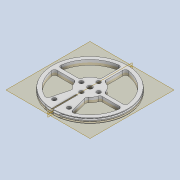
# Autodesk Inventor part: driver_wheel_1
Saved by Autodesk Inventor 2020 (Build 240168000, 168)
## iProperties
Created: 2021-08-04
Part Number: driver_wheel_1
Material: Generic
Document SubType Name: Modeling
Designer: Shuang Peng
Density: 1 g/cm^3
Appearance: Default
Author: Shuang Peng
Autodesk Inventor part; units mm, degrees
ref_plane "YZ Plane" through (0, 0, 0) normal (1, 0, 0) x (0, 1, 0)
ref_plane "XZ Plane" through (0, 0, 0) normal (0, 1, 0) x (-1, 0, 0)
ref_plane "XY Plane" through (0, 0, 0) normal (0, 0, 1) x (1, 0, 0)
sketch "Sketch1" plane through (0, 0, 0) normal (0, 1, 0) x (-1, 0, 0)
  circle A0 centre (0, 0) radius 30
  dimension "d0" = 60
  constraints: 1 centre point, 1 coincident
  measures "d0" diameter of A0
extrude "Extrusion1" add sketch "Sketch1" along normal blind 2
sketch "Sketch2" plane through (0, 0, 0) normal (1, 0, 0) x (0, 1, 0)
  line L0 (0, 30) -> (2, 30) projected
  line L1 (2, -30) -> (2, 30) projected
  line L2 (2, 30) -> (2, 31)
  line L3 (2, 31) -> (1, 30)
  line L4 (0, -30) -> (0, 30) projected
  line L5 (0, 30) -> (0, 31)
  line L6 (0, 31) -> (1, 30)
  line L7 (0, 0) -> (2, 0)
  dimension "d3" = 1
  dimension "d4" = 1
  constraints: 10 end point, 2 midpoint, 2 vertical
  measures "d3" distance of L0.end L2.end
  measures "d4" distance of L0.start L5.end
revolve "Revolution1" add sketch "Sketch2" angle 360 about axis through (0, 0, 0) along (0, 1, 0) contours L5 L6 L0 | L3 L2 L0
sketch "Sketch3" plane through (0, 2, 0) normal (0, 1, 0) x (1, 0, 0)
  circle A0 centre (0, 0) radius 1.5
  dimension "d6" = 3
  constraints: 1 centre point, 1 coincident
  measures "d6" diameter of A0
extrude "Extrusion2" cut sketch "Sketch3" against normal blind 2
sketch "Sketch4" plane through (0, 2, 0) normal (0, 1, 0) x (1, 0, 0)
  circle A0 centre (0, 0) radius 1.5 projected
  circle A1 centre (0, 0) radius 31 projected
  circle A2 centre (0, 0) radius 1.5 projected
  line L0 (0, 0) -> (0, -31)
  circle A3 centre (0, 0) radius 31 projected
  line L1 (0, -51) -> (0, -11) construction
  line L2 (0.5, -51) -> (0.5, -11)
  line L3 (-0.5, -11) -> (-0.5, -51)
  arc A4 (-0.5, -51) -> (0.5, -51) centre (0, -51) ccw
  arc A5 (0.5, -11) -> (-0.5, -11) centre (0, -11) ccw
  point P0 (-0.5, -30.996)
  point P1 (0.5, -30.996)
  dimension "d9" = 20
  dimension "d10" = 1
  constraints: 10 end point, 4 point on circle, 4 tangent, 2 centre point, 1 midpoint, 1 parallel, 1 point on line, 1 vertical, 1 vertical alignment, 1 other
  measures "d9" distance of L0.end L1.end
  measures "d10" diameter of A5
extrude "Extrusion3" cut sketch "Sketch4" against normal blind 2 contours L3 A5 L0 A1 | A1 L0 A5 L2
ref_plane "Work Plane1" through (0, 2, 30.996) normal (1, 0, 0) x (0, 0, -1)
sketch "Sketch5" plane through (-0.5, 2, 30.996) normal (1, 0, 0) x (0, 0, -1)
  line L0 (0, -2) -> (1.0001, -1) projected
  line L1 (19.996, -2) -> (0, -2) projected
  line L2 (19.996, 0) -> (19.996, -2) projected
  line L3 (0, 0) -> (19.996, 0) projected
  line L4 (1.0001, -1) -> (0, 0) projected
  line L5 (60.996, -1) -> (1.0001, -1) projected
  line L6 (1.0001, -1) -> (2.0001, -1)
  line L7 (0, 0) -> (19.996, 0) projected
  line L8 (2.0001, -1) -> (0, 0)
  line L9 (19.996, -2) -> (0, -2) projected
  line L10 (2.0001, -1) -> (0, -2)
  point P0 (30.996, -2)
  dimension "d13" = 1
  constraints: 6 end point, 1 parallel
  measures "d13" distance of L0.end L6.end
extrude "Extrusion4" cut sketch "Sketch5" against normal blind 12 contours L0 L5 L10 | L4 L8 L5
mirror "Mirror1" about plane through (0, 2, 30.996) normal (1, 0, 0) of "Extrusion4"
sketch "Sketch6" plane through (0, 2, 0) normal (0, 1, 0) x (1, 0, 0)
  line L0 (0.5, -11) -> (0.5, -30.996) projected
  arc A0 (0.5, -30.996) -> (-0.5, -30.996) centre (0, 0) ccw projected
  line L1 (-0.5, -30.996) -> (-0.5, -11) projected
  arc A1 (0.5, -11) -> (-0.5, -11) centre (0, -11) ccw projected
  circle A2 centre (0, 0) radius 1.5 projected
  line L2 (0, 0) -> (-6, 0)
  line L3 (-6, 0) -> (-6, -23)
  circle A3 centre (-6, -23) radius 1.6
  dimension "d16" = 6
  dimension "d17" = 23
  dimension "d18" = 3.2
  constraints: 4 end point, 1 centre point, 1 coincident, 1 horizontal, 1 perpendicular
  measures "d16" distance of L2.start L2.end
  measures "d17" distance of L2.end L3.end
  measures "d18" diameter of A3
extrude "Extrusion5" cut sketch "Sketch6" against normal blind 12 contours A3
mirror "Mirror2" about plane through (0, 2, 30.996) normal (1, 0, 0) of "Extrusion5"
ref_plane "Work Plane2" through (0, 2, 0) normal (0, 1, 0) x (1, 0, 0)
mirror "Mirror3" about plane through (0, 2, 0) normal (0, 1, 0) of "Extrusion1", "Revolution1", "Extrusion2", "Extrusion3", "Extrusion4", "Mirror1", "Extrusion5", "Mirror2"
chamfer "Chamfer1" distance 0.5 angle 45 3 edges at (0, 2, -31) (0, 4, -31) (0, 0, -31)
sketch "Sketch7" plane through (0, 4, 0) normal (0, 1, 0) x (1, 0, 0)
  line L0 (0, 0) -> (-7, 0)
  circle A0 centre (-7, 0) radius 1.6
  circle A1 centre (0, -7) radius 1.6
  circle A2 centre (7, 0) radius 1.6
  circle A3 centre (0, 7) radius 1.6
  dimension "d25" = 7
  dimension "d26" = 3.2
  dimension "d29" = 360
  constraints: 4 centre point, 2 end point, 1 coincident, 1 horizontal, 9 other
  measures "d25" distance of L0.start L0.end
  measures "d26" diameter of A0
extrude "Extrusion6" cut sketch "Sketch7" against normal blind 12
sketch "Sketch8" plane through (0, 4, 0) normal (0, 1, 0) x (1, 0, 0)
  circle A0 centre (7, 0) radius 1.6 projected
  circle A1 centre (0, 7) radius 1.6 projected
  circle A2 centre (0, -7) radius 1.6 projected
  circle A3 centre (-7, 0) radius 1.6 projected
  arc A4 (0.5, -30.4959) -> (-0.5, -30.4959) centre (0, 0) ccw projected
  line L0 (-0.5, -30.4959) -> (-0.5, -11) projected
  arc A5 (0.5, -11) -> (-0.5, -11) centre (0, -11) ccw projected
  line L1 (0.5, -11) -> (0.5, -30.4959) projected
  circle A6 centre (6, -23) radius 1.6 projected
  circle A7 centre (-6, -23) radius 1.6 projected
  circle A8 centre (0, 0) radius 1.5 projected
  circle A9 centre (0, 0) radius 1.5 projected
  circle A10 centre (0, 0) radius 10
  circle A11 centre (0, 0) radius 27.5
  line L2 (0, 0) -> (-27.5, 0)
  line L3 (-9.8869, -1.5) -> (-27.4591, -1.5)
  line L4 (0, 0) -> (-6, -23)
  line L5 (-5.3108, -8.4732) -> (-9.803, -25.6934)
  line L6 (0, 0) -> (0, 27.5)
  line L7 (-9.8869, 1.5) -> (-27.4591, 1.5)
  line L8 (-1.5, 9.8869) -> (-1.5, 27.4591)
  dimension "d33" = 20
  dimension "d34" = 55
  dimension "d35" = 3
  dimension "d36" = 1.5
  dimension "d37" = 1.5
  dimension "d38" = 1.5
  constraints: 14 end point, 10 point on circle, 4 parallel, 2 centre point, 2 coincident, 1 horizontal, 1 vertical
  measures "d33" diameter of A10
  measures "d34" diameter of A11
  measures "d35" distance between parallel lines of L4 L5
  measures "d36" distance between parallel lines of L2 L3
  measures "d37" distance between parallel lines of L2 L7
  measures "d38" distance between parallel lines of L6 L8
extrude "Extrusion7" cut sketch "Sketch8" against normal blind 12 contours A10 L7 A11 L8 | L5 A11 L3 A10
mirror "Mirror4" about plane through (0, 2, 30.996) normal (-1, 0, 0) of "Extrusion7"
fillet "Fillet1" radius 2 8 edges at (-9.803, 2, 25.6934) (-27.4591, 2, 1.5) (-27.4591, 2, -1.5) (-1.5, 2, -27.4591) (-1.5, 2, -9.8869) (-9.8869, 2, -1.5) (-9.8869, 2, 1.5) (-5.3108, 2, 8.4732)
mirror "Mirror5" about plane through (0, 2, 30.996) normal (1, 0, 0) of "Fillet1"
chamfer "Chamfer2" distance 0.5 angle 45 2 edges at (-1.5, 4, 0) (-1.5, 0, 0)
ref_plane "Work Plane3" through (0, 2, 30.996) normal (-1, 0, 0) x (0, 0, -1)
body "Solid1"
